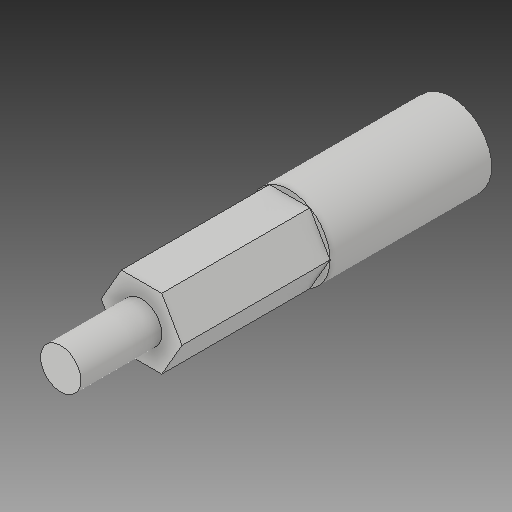
# Autodesk Inventor part: Front_Wheel_Attachment
Saved by Autodesk Inventor 2019 (Build 230136000, 136)
## iProperties
Created: 2019-03-03
Part Number: Front_Wheel_Attachment
Material: Generic
Document SubType Name: Modeling
Designer: alarr
Density: 1 g/cm^3
Appearance: Default
Author: alarr
Autodesk Inventor part; units mm, degrees
ref_plane "YZ Plane" through (0, 0, 0) normal (1, 0, 0) x (0, 1, 0)
ref_plane "XZ Plane" through (0, 0, 0) normal (0, 1, 0) x (-1, 0, 0)
ref_plane "XY Plane" through (0, 0, 0) normal (0, 0, 1) x (1, 0, 0)
sketch "Sketch1" plane through (0, 0, 0) normal (0, 0, 1) x (1, 0, 0)
  circle A0 centre (0, 0) radius 3.81 projected
  circle A1 centre (0, 0) radius 3.81
  point P0 (0, 0)
  constraints: 1 centre point, 1 coincident, 1 concentric
extrude "Extrusion1" add sketch "Sketch1" against normal blind 12.7
sketch "Sketch2" plane through (0, 0, 0) normal (0, 0, 1) x (1, 0, 0)
  circle A0 centre (0, 0) radius 3.81 projected
  circle A1 centre (0, 0) radius 3.81
  point P0 (0, 0)
  constraints: 1 centre point, 1 coincident, 1 concentric
extrude "Extrusion2" add sketch "Sketch2" along normal blind 2.54
sketch "Sketch3" plane through (0, 0, 2.54) normal (0, 0, 1) x (1, 0, 0)
  circle A0 centre (0, 0) radius 3.81 projected
  line L0 (-1.905, -3.2996) -> (-3.81, 0)
  line L1 (-3.81, 0) -> (-1.905, 3.2996)
  line L2 (-1.905, 3.2996) -> (1.905, 3.2996)
  line L3 (1.905, 3.2996) -> (3.81, 0)
  line L4 (3.81, 0) -> (1.905, -3.2996)
  line L5 (1.905, -3.2996) -> (-1.905, -3.2996)
  point P0 (0, 0)
  point P1 (0, 0)
  constraints: 12 end point, 1 coincident, 1 horizontal, 15 other
extrude "Extrusion3" add sketch "Sketch3" along normal blind 13.97 contours L4 L5 L0 L1 L2 L3
sketch "Sketch4" plane through (0, 0, 16.51) normal (0, 0, 1) x (1, 0, 0)
  circle A0 centre (0, 0) radius 1.905
  dimension "d6" = 3.81
  constraints: 1 centre point, 1 coincident
  measures "d6" diameter of A0
extrude "Extrusion4" add sketch "Sketch4" along normal blind 7.62
body "Solid1"
